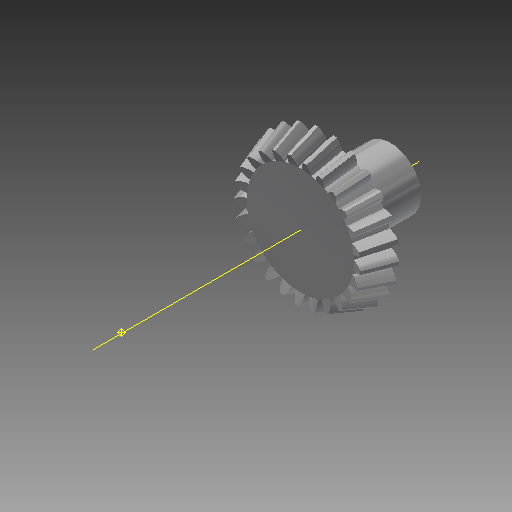
# Autodesk Inventor part: Bevel Gear1
Saved by Autodesk Inventor 2019 (Build 230136000, 136)
## iProperties
Created: 2019-11-21
Part Number: Bevel Gear1
Material: Steel, Mild
Document SubType Name: Modeling
Designer: felix
Categories: <?xml version="1.0" encoding="UTF-16"?> <MemberInstance><Categories><FamilyTemplate><FamilyTemplateParameter ValueType="xs:double" Id="1" ObjectReferenceKey="da_z" ObjectType="kUserParameterObject"/><FamilyTemplateParameter ValueType="xs:double" Id="2" ObjectReferenceKey="da_b" ObjectType="kUserParameterObject"/><FamilyTemplateParameter ValueType="xs:double" Id="3" ObjectReferenceKey="da_beta" ObjectType="kUserParameterObject"/><FamilyTemplateParameter ValueType="xs:double" Id="4" ObjectReferenceKey="da_dae" ObjectType="kUserParameterObject"/><FamilyTemplateParameter ValueType="xs:double" Id="5" ObjectReferenceKey="da_ve" ObjectType="kUserParameterObject"/><FamilyTemplateParameter ValueType="xs:double" Id="6" ObjectReferenceKey="da_omega" ObjectType="kUserParameterObject"/><FamilyTemplateParameter ValueType="xs:string" Id="7" ObjectReferenceKey="EAIAABAAAAAAHwAAAAAAAIAAAAAAAAAA" ObjectType="83914240" SubObjectId="SurfaceGeometry"/></FamilyTemplate><ParamToTemplateMap><ParamToTemplate CategoryParameter="//CategoryParameter[@InternalName='046C89C9-8512-4d59-83FE-43B91F4F132A']" TemplateParameter="1"/><ParamToTemplate CategoryParameter="//CategoryParameter[@InternalName='2552DF32-E462-4b46-AEBF-C6C7768E72AC']" TemplateParameter="2"/><ParamToTemplate CategoryParameter="//CategoryParameter[@InternalName='C9EE641D-15FC-4fae-A226-E94C4372FDD7']" TemplateParameter="3"/><ParamToTemplate><ParamToTemplate CategoryParameter="//CategoryParameter[@InternalName='00B6519A-459B-49c7-AD84-2E56D39A5744']" ConstantValue="0.000000"/></ParamToTemplate><ParamToTemplate><ParamToTemplate CategoryParameter="//CategoryParameter[@InternalName='04B31F0E-C7A6-4894-AA32-9629BEFACF47']" ConstantValue="1.000000"/></ParamToTemplate><ParamToTemplate><ParamToTemplate CategoryParameter="//CategoryParameter[@InternalName='43CBEC2E-7847-49e7-A936-2F7889FCB2D9']" ConstantValue="0.200000"/></ParamToTemplate><ParamToTemplate><ParamToTemplate CategoryParameter="//CategoryParameter[@InternalName='B1EFC894-105D-4ebd-86BF-FA20ED196853']" ConstantValue="0.300000"/></ParamToTemplate><ParamToTemplate><ParamToTemplate CategoryParameter="//CategoryParameter[@InternalName='51175063-3D10-4879-93E8-6246FE8B403D']" ConstantValue="2060000000.000000"/></ParamToTemplate><ParamToTemplate><ParamToTemplate CategoryParameter="//CategoryParameter[@InternalName='A3A52E27-4454-46a9-B0BD-C932399B70AF']" ConstantValue="0.300000"/></ParamToTemplate><ParamToTemplate CategoryParameter="//CategoryParameter[@InternalName='2A200944-5A8C-41ca-B96E-8520D2E510F1']" TemplateParameter="4"/><ParamToTemplate><ParamToTemplate CategoryParameter="//CategoryParameter[@InternalName='1A637F62-92C8-44bc-B81F-10802510B579']" ConstantValue="20.805352"/></ParamToTemplate><ParamToTemplate CategoryParameter="//CategoryParameter[@InternalName='B52DD4BE-6863-48fb-BF58-89EF6F9EC65C']" TemplateParameter="5"/><ParamToTemplate><ParamToTemplate CategoryParameter="//CategoryParameter[@InternalName='3956BFF2-84D2-457d-93C2-9B0613DEBA67']" ConstantValue="28.761979"/></ParamToTemplate><ParamToTemplate CategoryParameter="//CategoryParameter[@InternalName='739CFA02-461B-4bf8-8049-181FCAD8B28F']" TemplateParameter="6"/><ParamToTemplate><ParamToTemplate CategoryParameter="//CategoryParameter[@InternalName='A27E999F-E2CE-4481-8A2A-EBF499C4C3C5']" ConstantValue="0.000000"/></ParamToTemplate><ParamToTemplate><ParamToTemplate CategoryParameter="//CategoryParameter[@InternalName='9E1B4470-B2D3-4ff1-B813-535BB4CDF51A']" ConstantValue="3520000.000000"/></ParamToTemplate><ParamToTemplate><ParamToTemplate CategoryParameter="//CategoryParameter[@InternalName='F8452263-BFF6-458c-9FB1-07C4B99E95CD']" ConstantValue="11400000.000000"/></ParamToTemplate><ParamToTemplate><ParamToTemplate CategoryParameter="//CategoryParameter[@InternalName='3E3BB259-FD49-497f-8171-6EBC954A3479']" ConstantValue="2.000000"/></ParamToTemplate><ParamToTemplate CategoryParameter="//CategoryParameter[@InternalName='27C3BAF2-7550-4e4b-AE2C-0DB134B7D9B7']" TemplateParameter="7"/></ParamToTemplateMap><Category DisplayName="Gear" InternalName="DC85795E-93AB-48d5-8EEE-5A27447B64BD" Mnemonic="Gear"><CategoryParameter DisplayName="z" InternalName="046C89C9-8512-4d59-83FE-43B91F4F132A" Mnemonic="z"/><CategoryParameter DisplayName="b" InternalName="2552DF32-E462-4b46-AEBF-C6C7768E72AC" Mnemonic="b"/><CategoryParameter DisplayName="||b|" InternalName="C9EE641D-15FC-4fae-A226-E94C4372FDD7" Mnemonic="beta"/><CategoryParameter DisplayName="x" InternalName="00B6519A-459B-49c7-AD84-2E56D39A5744" Mnemonic="x"/><CategoryParameter DisplayName="a*" InternalName="04B31F0E-C7A6-4894-AA32-9629BEFACF47" Mnemonic="a"/><CategoryParameter DisplayName="c*" InternalName="43CBEC2E-7847-49e7-A936-2F7889FCB2D9" Mnemonic="c"/><CategoryParameter DisplayName="r|.f|*" InternalName="B1EFC894-105D-4ebd-86BF-FA20ED196853" Mnemonic="rf"/><CategoryParameter DisplayName="E" InternalName="51175063-3D10-4879-93E8-6246FE8B403D" Mnemonic="E"/><CategoryParameter DisplayName="||m|" InternalName="A3A52E27-4454-46a9-B0BD-C932399B70AF" Mnemonic="mi"/><Category DisplayName="BevelGear" InternalName="0C98F69A-0C2B-4791-B2FE-7691BB227E77" Mnemonic="BevelGear"><CategoryParameter DisplayName="d|.ae|" InternalName="2A200944-5A8C-41ca-B96E-8520D2E510F1" Mnemonic="dae"/><CategoryParameter DisplayName="d|.ai|" InternalName="1A637F62-92C8-44bc-B81F-10802510B579" Mnemonic="dai"/><CategoryParameter DisplayName="A|.e|" InternalName="B52DD4BE-6863-48fb-BF58-89EF6F9EC65C" Mnemonic="ve"/><CategoryParameter DisplayName="A|.i|" InternalName="3956BFF2-84D2-457d-93C2-9B0613DEBA67" Mnemonic="vi"/><CategoryParameter DisplayName="||S|" InternalName="739CFA02-461B-4bf8-8049-181FCAD8B28F" Mnemonic="omega"/><CategoryParameter DisplayName="x|.t|" InternalName="A27E999F-E2CE-4481-8A2A-EBF499C4C3C5" Mnemonic="xt"/><CategoryParameter DisplayName="||s||.Flim|" InternalName="9E1B4470-B2D3-4ff1-B813-535BB4CDF51A" Mnemonic="sFlim"/><CategoryParameter DisplayName="||s||.Hlim|" InternalName="F8452263-BFF6-458c-9FB1-07C4B99E95CD" Mnemonic="sHlim"/><CategoryParameter DisplayName="type" InternalName="3E3BB259-FD49-497f-8171-6EBC954A3479" Mnemonic="type"/><CategoryParameter DisplayName="PitchDiameter" InternalName="27C3BAF2-7550-4e4b-AE2C-0DB134B7D9B7" Mnemonic="IDS_PITCHDIAM"/></Category></Category></Categories></MemberInstance>
Mass: 18543.9 g
Surface Area: 1741.34 cm^2
Volume: 2362.29 cm^3
Density: 7.85 g/cm^3
Appearance: Steel
CustomPartVersion: 1
Author: felix
Autodesk Inventor part; units mm, degrees
ref_plane "Mesh Plane2" through (0, 0, 0) normal (0.9921147, 0.1253332, 0) x (0, 0, 1)
sketch "Teeth Body Sketch" plane through (0, 0, 0) normal (1, 0, 0) x (0, 1, 0)
  line L0 (0, 0) -> (102.25422, -340.91526) construction
  line L1 (102.25422, -340.91526) -> (121.03815, -334.65395)
  line L2 (121.03815, -334.65395) -> (0, 0) construction
  line L3 (112.5, -337.5) -> (0, 0) construction
  line L4 (87.882832, -293.001095) -> (104.026761, -287.619785)
  line L5 (102.25422, -340.91526) -> (87.882832, -293.001095)
  line L6 (121.03815, -334.65395) -> (104.026761, -287.619785)
  line L7 (0, -39.386751) -> (0, 6.564458)
  line L8 (0, -337.5) -> (121.03815, -337.5) construction
  dimension "d0" = 225
  dimension "d1" = 204.50844
  dimension "d2" = 242.0763
  dimension "d3" = 50
  dimension "d4" = 334.65395
  constraints: 16 end point, 4 point on line, 3 perpendicular, 2 collinear, 1 horizontal alignment, 1 vertical alignment
  measures "d0" diameter of L3.start L7
  measures "d1" diameter of L0.end L7
  measures "d2" diameter of L1.end L7
  measures "d3" distance between parallel lines of L1 L4
  measures "d4" vertical distance of L1.end L0.start
revolve "Teeth Body" add sketch "Teeth Body Sketch" angle 360 about axis through (0, 0, 0) along (0, 0, 1)
ref_plane "Tooth Plane" through (0, 112.5, -337.5) normal (0, -0.3162278, 0.9486833) x (1, 0, 0)
sketch "Start Sketch" plane through (0, 112.5, -337.5) normal (0, -0.3162278, 0.9486833) x (1, 0, 0)
  line L0 (0, -23.505131) -> (0, 10.644758)
  arc A0 (-3.67457, -13.176) -> (-17.063661, 13.8452) centre (-47.040386, -17.836132) ccw
  arc A1 (17.063661, 13.8452) -> (3.67457, -13.176) centre (47.040386, -17.836132) ccw
  line L1 (-3.67457, -13.176) -> (3.67457, -13.176)
  arc A2 (17.063661, 13.8452) -> (-17.063661, 13.8452) centre (0, -118.585412) ccw
  dimension "d7" = 43.61549
  dimension "d8" = 47.04039
  dimension "d9" = 100.74928
  dimension "d57" = 133.52541
  dimension "d58" = 105.40941
  constraints: 6 point on circle, 3 centre point, 3 symmetric about line, 2 end point, 1 coincident, 1 perpendicular, 1 other
  measures "d7" radius of A0
  measures "d8" horizontal distance of point (0, -118.585) A0.centre
  measures "d9" vertical distance of point (0, -118.585) A0.centre
  measures "d57" radius of A2
  measures "d58" distance from line of A2.centre L1
sketch "End Sketch" plane through (0, 96.375546, -289.126639) normal (0, -0.3162278, 0.9486833) x (1, 0, 0)
  line L0 (0, -15.358918) -> (0, 6.982715)
  arc A0 (-3.151574, -11.182095) -> (-14.635016, 11.99322) centre (-40.3452, -15.178957) ccw
  arc A1 (14.635016, 11.99322) -> (3.151574, -11.182095) centre (40.3452, -15.178957) ccw
  line L1 (-3.151574, -11.182095) -> (3.151574, -11.182095)
  arc A2 (14.635016, 11.99322) -> (-14.635016, 11.99322) centre (0, -101.588746) ccw
  dimension "d12" = 37.40776
  dimension "d15" = 40.3452
  dimension "d16" = 86.40979
  dimension "d59" = 114.52094
  dimension "d60" = 90.40665
  constraints: 6 point on circle, 3 centre point, 3 symmetric about line, 2 end point, 1 coincident, 1 other
  measures "d12" radius of A0
  measures "d15" horizontal distance of A0.centre point (0, -101.589)
  measures "d16" vertical distance of A0.centre point (0, -101.589)
  measures "d59" radius of A2
  measures "d60" distance from line of A2.centre L1
loft "Loft" cut profiles "Start Sketch", "End Sketch"
pattern_circular "Circular Pattern" count 25 over 360 about axis through (0, 0, 0) along (0, 0, 1) of "Loft"
ref_plane "End Plane" through (0, 96.375546, -289.126639) normal (0, -0.3162278, 0.9486833) x (1, 0, 0)
sketch3d "3D Sketch Right"
ref_plane "End Plane Right" through (-17.010945, 94.862393, -289.126639) normal (0.0558164, -0.3112628, 0.9486833) x (0.9842994, 0.1765069, 0)
sketch "End Sketch Right" plane through (-17.010945, 94.862393, -289.126639) normal (0.0558164, -0.3112628, 0.9486833) x (0.9842994, 0.1765069, 0)
  arc A0 (-3.151574, -11.182095) -> (-14.635016, 11.99322) centre (-40.3452, -15.178957) ccw
  line L0 (0, -125.709938) -> (0, 27.91224)
  arc A1 (14.635016, 11.99322) -> (3.151574, -11.182095) centre (40.3452, -15.178957) ccw
  line L1 (-3.151574, -11.182095) -> (3.151574, -11.182095)
  arc A2 (14.635016, 11.99322) -> (-14.635016, 11.99322) centre (0, -101.588746) ccw
  dimension "d70" = 40.3452
  dimension "d71" = 86.40979
  dimension "d72" = 37.40776
  dimension "d73" = 90.40665
  dimension "d74" = 114.52094
  constraints: 6 point on circle, 3 centre point, 3 symmetric about line, 2 end point, 1 coincident, 1 perpendicular, 1 other
  measures "d70" horizontal distance of A2.centre A0.centre
  measures "d71" vertical distance of point (0, -101.589) A0.centre
  measures "d72" radius of A0
  measures "d73" distance from line of point (0, -101.589) L1
  measures "d74" radius of A2
feature "Loft Right" [suppressed]
pattern_circular "Circular Pattern Right" [suppressed]
sketch3d "3D Sketch Left"
ref_plane "End Plane Left" through (16.93906, 94.862393, -289.10142) normal (-0.0555856, -0.3112913, 0.9486875) x (0.9844287, -0.1757841, 0)
sketch "End Sketch Left" plane through (16.93906, 94.862393, -289.10142) normal (-0.0555856, -0.3112913, 0.9486875) x (0.9844287, -0.1757841, 0)
  line L0 (0, -128.704549) -> (0, 30.913195)
  arc A0 (-3.151574, -11.178057) -> (-14.635016, 11.997257) centre (-40.3452, -15.174919) ccw
  arc A1 (14.635016, 11.997257) -> (3.151574, -11.178057) centre (40.3452, -15.174919) ccw
  line L1 (-3.151574, -11.178057) -> (3.151574, -11.178057)
  ellipse E0 centre (0, -90.949747) end of major axis (104.026761, -90.949747) minor radius 98.688887
  arc A2 (14.635016, 11.997257) -> (-14.635016, 11.997257) centre (0, -101.584708) ccw
  dimension "d56" = 98.68889
  dimension "d30" = 37.40776
  dimension "d31" = 40.3452
  dimension "d32" = 86.40979
  dimension "d61" = 114.52094
  dimension "d62" = 90.40665
  constraints: 6 point on circle, 3 centre point, 3 symmetric about line, 2 end point, 1 coincident, 2 other
  measures "d30" radius of A0
  measures "d31" horizontal distance of point (0, -101.585) A0.centre
  measures "d32" vertical distance of A0.centre point (0, -101.585)
  measures "d61" radius of A2
  measures "d62" distance from line of point (0, -101.585) L1
feature "Loft Left" [suppressed]
pattern_circular "Circular Pattern Left" [suppressed]
sketch "Body Sketch" plane through (0, 0, 0) normal (1, 0, 0) x (0, 1, 0)
  line L0 (0, -35.037536) -> (0, -19.530831)
  line L1 (102.25422, -340.91526) -> (87.882832, -293.001095)
  line L2 (87.882832, -293.001095) -> (0, -293.001095)
  line L3 (102.25422, -340.91526) -> (0, -340.91526)
  constraints: 4 end point, 2 perpendicular, 2 point on line
sketch "Body Sketch outline for Fix Body" plane through (0, 0, 0) normal (1, 0, 0) x (0, 1, 0)
  line L0 (0, -340.91526) -> (102.25422, -340.91526)
  line L1 (0, -293.001095) -> (0, -340.91526)
  line L2 (87.882832, -293.001095) -> (0, -293.001095)
  line L3 (102.25422, -340.91526) -> (87.882832, -293.001095)
revolve "Fix Body" add sketch "Body Sketch outline for Fix Body" angle 360 about axis through (0, 0, 0) along (0, 0, 1)
sketch "Sketch6" plane through (0, 0, 0) normal (1, 0, 0) x (0, 1, 0)
  line L0 (112.5, -337.5) -> (0, 0)
  line L1 (0, -37.799919) -> (0, 6.299986)
surface revolve "Pitch Diameter" sketch "Sketch6" angle 360 about axis through (0, 0, 0) along (0, 0, 1) shown no curves L0
sketch "Sketch8" plane through (0, 0, -340.91526) normal (0, 0, -1) x (-1, 0, 0)
  circle A0 centre (0, 0) radius 50
  dimension "d94" = 100
  constraints: 1 centre point, 1 coincident
  measures "d94" diameter of A0
extrude "Extrusion1" add sketch "Sketch8" along normal blind 100
sketch "Sketch9" plane through (0, 0, -440.91526) normal (0, 0, -1) x (-1, 0, 0)
  circle A0 centre (0, 0) radius 19
  dimension "d99" = 38
  constraints: 1 centre point, 1 coincident
  measures "d99" diameter of A0
extrude "Extrusion2" cut sketch "Sketch9" against normal blind 70
equation "\"d0\" = da_de"
equation "\"d1\" = da_dfe"
equation "\"d2\" = da_dae"
equation "\"d3\" = da_b"
equation "\"d4\" = da_ve"
equation "\"d7\" = fd_rr"
equation "\"d8\" = fd_x"
equation "\"d9\" = fd_y"
equation "\"d57\" = 0.5 * fd_dva + 0.3 * da_he"
equation "\"d58\" = 0.5 * fd_dva - 1.12 * da_he"
equation "\"da_teethtype\" = 0"
equation "\"da_b\" = 50"
equation "\"da_de\" = 225"
equation "\"da_dae\" = 242.0763"
equation "\"da_dfe\" = 204.50844"
equation "\"da_le\" = 355.75624"
equation "\"da_omega\" = 90deg"
equation "\"da_beta\" = 0"
equation "\"da_delta\" = 18.434949deg"
equation "\"da_alpha\" = 20deg"
equation "\"da_he\" = 19.8"
equation "\"da_ve\" = 334.65395"
equation "\"da_zv\" = 26.352314"
equation "\"fd_loft\" = da_b + 0.05 * da_he"
equation "\"fd_x\" = fd_x1 + fd_x2"
equation "\"fd_y\" = fd_y1 - fd_y2"
equation "\"fd_dd\" = fd_dva - 0.8 * da_he"
equation "\"da_dvw\" = 237.17082"
equation "\"d11\" = fd_loft"
equation "\"da_dm\" = 209.18861"
equation "\"da_x\" = 0"
equation "\"da_m\" = 9"
equation "\"d50\" = da_omega"
equation "\"fd_rr\" = 43.615489"
equation "\"fd_dva\" = 255.170825"
equation "\"fd_x1\" = 7.142797"
equation "\"fd_x2\" = 39.897589"
equation "\"fd_y1\" = 118.370099"
equation "\"fd_y2\" = 17.620819"
body "Solid1"
body "Srf1"
